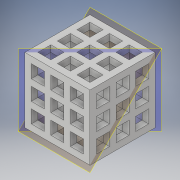
# Autodesk Inventor part: Probewürfel_Hydrogel
Saved by Autodesk Inventor 2018 (Build 220112000, 112)
## iProperties
Created: 2020-04-19
Part Number: Probewürfel_Hydrogel
Material: Generisch
Document SubType Name: Modeling
Designer: maxse
Density: 1 g/cm^3
Appearance: Vorgabe
Author: maxse
Autodesk Inventor part; units mm, degrees
ref_plane "YZ Plane" through (0, 0, 0) normal (1, 0, 0) x (0, 1, 0)
ref_plane "XZ Plane" through (0, 0, 0) normal (0, 1, 0) x (-1, 0, 0)
ref_plane "XY Plane" through (0, 0, 0) normal (0, 0, 1) x (1, 0, 0)
sketch "Skizze1" plane through (0, 0, 0) normal (0, 1, 0) x (-1, 0, 0)
  line L0 (0, 0) -> (10, 0)
  line L1 (10, 0) -> (10, -10)
  line L2 (10, -10) -> (0, -10)
  line L3 (0, -10) -> (0, 0)
  dimension "d0" = 10
  dimension "d1" = 10
  constraints: 8 end point, 2 parallel, 1 horizontal, 1 perpendicular
  measures "d0" distance of L1.end L2.end
  measures "d1" distance of L0.end L1.end
extrude "Extrusion1" add sketch "Skizze1" along normal blind 10
sketch "Skizze2" plane through (-10, 0, 0) normal (0, 0, 1) x (1, 0, 0)
  line L0 (1, 9) -> (3, 9)
  line L1 (3, 9) -> (3, 7)
  line L2 (3, 7) -> (1, 7)
  line L3 (1, 7) -> (1, 9)
  line L4 (0, 10) -> (10, 10) projected
  line L5 (0, 0) -> (0, 10) projected
  line L6 (1, 6) -> (3, 6)
  line L7 (3, 6) -> (3, 4)
  line L8 (3, 4) -> (1, 4)
  line L9 (1, 4) -> (1, 6)
  line L10 (1, 3) -> (3, 3)
  line L11 (3, 3) -> (3, 1)
  line L12 (3, 1) -> (1, 1)
  line L13 (1, 1) -> (1, 3)
  line L14 (4, 9) -> (6, 9)
  line L15 (6, 9) -> (6, 7)
  line L16 (6, 7) -> (4, 7)
  line L17 (4, 7) -> (4, 9)
  line L18 (4, 6) -> (6, 6)
  line L19 (6, 6) -> (6, 4)
  line L20 (6, 4) -> (4, 4)
  line L21 (4, 4) -> (4, 6)
  line L22 (4, 3) -> (6, 3)
  line L23 (6, 3) -> (6, 1)
  line L24 (6, 1) -> (4, 1)
  line L25 (4, 1) -> (4, 3)
  line L26 (7, 9) -> (9, 9)
  line L27 (9, 9) -> (9, 7)
  line L28 (9, 7) -> (7, 7)
  line L29 (7, 7) -> (7, 9)
  line L30 (7, 6) -> (9, 6)
  line L31 (9, 6) -> (9, 4)
  line L32 (9, 4) -> (7, 4)
  line L33 (7, 4) -> (7, 6)
  line L34 (7, 3) -> (9, 3)
  line L35 (9, 3) -> (9, 1)
  line L36 (9, 1) -> (7, 1)
  line L37 (7, 1) -> (7, 3)
  line L38 (10, 0) -> (0, 0) projected
  dimension "d4" = 2
  dimension "d5" = 2
  dimension "d6" = 1
  dimension "d7" = 1
  dimension "d8" = 2
  dimension "d9" = 2
  dimension "d10" = 2
  dimension "d11" = 2
  dimension "d12" = 2
  dimension "d13" = 2
  dimension "d14" = 1
  dimension "d15" = 1
  dimension "d16" = 1
  dimension "d17" = 1
  dimension "d18" = 1
  dimension "d19" = 1
  dimension "d20" = 1
  dimension "d21" = 1
  dimension "d22" = 1
  dimension "d23" = 2
  dimension "d24" = 1
  dimension "d25" = 2
  constraints: 72 end point, 18 parallel, 14 point on line, 9 horizontal, 9 perpendicular
  measures "d4" distance of L1.end L2.end
  measures "d5" distance of L0.end L1.end
  measures "d6" distance between parallel lines of L4 L0
  measures "d7" distance between parallel lines of L5 L3
  measures "d8" distance of L6.end L7.end
  measures "d9" distance of L10.end L11.end
  measures "d10" distance of L15.end L16.end
  measures "d11" distance of L18.end L19.end
  measures "d12" distance of L27.end L28.end
  measures "d13" distance of L26.end L27.end
  measures "d14" distance between parallel lines of L6 L2
  measures "d15" distance between parallel lines of L10 L8
  measures "d16" distance between parallel lines of L4 L14
  measures "d17" distance between parallel lines of L1 L17
  measures "d18" distance between parallel lines of L29 L15
  measures "d19" distance between parallel lines of L30 L28
  measures "d20" distance between parallel lines of L4 L26
  measures "d21" distance between parallel lines of L34 L32
  measures "d22" distance between parallel lines of L38 L36
  measures "d23" distance of L30.end L31.end
  measures "d24" distance between parallel lines of L5 L13
  measures "d25" distance of L11.end L12.end
extrude "Extrusion2" cut sketch "Skizze2" against normal blind 10
ref_plane "Arbeitsebene2" through (-10, 10, 0) normal (0, -0.7071, 0.7071) x (0, -0.7071, -0.7071)
mirror "Spiegeln1" about plane through (-10, 10, 0) normal (0, -0.7071, 0.7071) of "Extrusion2"
ref_plane "Arbeitsebene3" through (0, 10, -10) normal (-0.7071, 0.7071, 0) x (-0.7071, -0.7071, 0)
mirror "Spiegeln2" about plane through (0, 10, -10) normal (-0.7071, 0.7071, 0) of "Extrusion2", "Spiegeln1"
